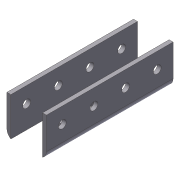
# Autodesk Inventor part: Frame_OuterConveyorMount
Saved by Autodesk Inventor 2012 (Build 160160000, 160)
## iProperties
Created: 2012-01-13
Part Number: Frame_OuterConveyorMount
Material: Aluminum-6061
Document SubType Name: Modeling
Designer: JesseK
Density: 2.71 g/cm^3
Mass: 57.9828 g
Surface Area: 157.919 cm^2
Volume: 21.3958 cm^3
Author: JesseK
Autodesk Inventor part; units mm, degrees
ref_plane "YZ Plane" through (0, 0, 0) normal (1, 0, 0) x (0, 1, 0)
ref_plane "XZ Plane" through (0, 0, 0) normal (0, 1, 0) x (-1, 0, 0)
ref_plane "XY Plane" through (0, 0, 0) normal (0, 0, 1) x (1, 0, 0)
sketch "Sketch1" plane through (0, 0, 0) normal (0, 0, 1) x (1, 0, 0)
  line L0 (0, 25.4) -> (0, 0)
  line L1 (6.35, -6.35) -> (25.4, -6.35)
  line L2 (31.75, 0) -> (31.75, 25.4)
  line L3 (31.75, 25.4) -> (28.575, 25.4)
  line L4 (28.575, 25.4) -> (28.575, 0)
  line L5 (25.4, -3.175) -> (6.35, -3.175)
  line L6 (3.175, 0) -> (3.175, 25.4)
  line L7 (3.175, 25.4) -> (0, 25.4)
  arc A0 (3.175, 0) -> (6.35, -3.175) centre (6.35, 0) ccw
  arc A1 (0, 0) -> (6.35, -6.35) centre (6.35, 0) ccw
  arc A2 (25.4, -3.175) -> (28.575, 0) centre (25.4, 0) ccw
  arc A3 (25.4, -6.35) -> (31.75, 0) centre (25.4, 0) ccw
  dimension "d0" = 3.175
  dimension "d1" = 25.4
  dimension "d2" = 25.4
  dimension "d3" = 3.175
  constraints: 17 end point, 8 point on circle, 8 tangent, 4 centre point, 4 horizontal, 4 vertical, 2 concentric, 1 coincident, 1 equal radius, 1 parallel
  measures "d0" distance between parallel lines of L6 L0
  measures "d1" distance of L6.start L6.end
  measures "d2" distance between parallel lines of L4 L6
  measures "d3" radius of A0
extrude "Extrusion1" add sketch "Sketch1" along normal blind 101.6
sketch "Sketch2" plane through (31.75, 0, 0) normal (1, 0, 0) x (0, 0, -1)
  line L0 (-101.6, 25.4) -> (-101.6, 0) projected
  line L1 (0, 25.4) -> (-101.6, 25.4) projected
  circle A0 centre (-88.9, 12.7) radius 3.175
  dimension "d6" = 6.35
  dimension "d7" = 12.7
  dimension "d8" = 12.7
  constraints: 1 centre point
  measures "d6" diameter of A0
  measures "d7" distance from line of L0 A0.centre
  measures "d8" distance from line of L1 A0.centre
extrude "Extrusion2" cut sketch "Sketch2" against normal through all
pattern_linear "Rectangular Pattern1" count 7 spacing 25.4 along (0, 0, -1) of "Extrusion2"
sketch "Sketch3" plane through (6.35, -6.35, 0) normal (0, -1, 0) x (1, 0, 0)
  line L0 (19.05, 101.6) -> (0, 101.6) projected
  circle A0 centre (9.525, 50.8) radius 6.35
  point P0 (-6.35, 0)
  dimension "d14" = 12.7
  dimension "d15" = 50.8
  constraints: 1 centre point
  measures "d14" diameter of A0
  measures "d15" distance from line of L0 A0.centre
extrude "Extrusion3" cut sketch "Sketch3" against normal up to next
sketch "Sketch4" plane through (6.35, -6.35, 0) normal (0, -1, 0) x (1, 0, 0)
  line L0 (19.05, 101.6) -> (0, 101.6) projected
  line L1 (0, 0) -> (0, 101.6) projected
  line L2 (0, 0) -> (19.05, 0) projected
  line L3 (19.05, 0) -> (19.05, 101.6) projected
  line L4 (-3.175, 101.6) -> (22.225, 101.6)
  line L5 (22.225, 101.6) -> (22.225, 73.025)
  line L6 (22.225, 73.025) -> (-3.175, 73.025)
  line L7 (-3.175, 73.025) -> (-3.175, 101.6)
  line L8 (-3.175, 165.9576) -> (0, 165.9576) construction
  line L9 (19.05, 165.9576) -> (22.225, 165.9576) construction
  line L10 (-3.175, 0) -> (22.225, 0)
  line L11 (22.225, 0) -> (22.225, 28.575)
  line L12 (22.225, 28.575) -> (-3.175, 28.575)
  line L13 (-3.175, 28.575) -> (-3.175, 0)
  line L14 (-6.35, 101.6) -> (-3.175, 101.6)
  line L15 (-3.175, 101.6) -> (-3.175, 73.025)
  line L16 (-3.175, 73.025) -> (-6.35, 73.025)
  line L17 (-6.35, 73.025) -> (-6.35, 101.6)
  point P0 (-6.35, 0)
  dimension "d18" = 25.4
  dimension "d19" = 28.575
  dimension "d20" = 0
  dimension "d21" = 0
  constraints: 28 end point, 6 parallel, 5 horizontal, 4 collinear, 4 point on line, 3 perpendicular
  measures "d18" distance of L5.end L6.end
  measures "d19" distance of L6.end L4.start
  measures "d20" distance between parallel lines of L0 L4
  measures "d21" distance between parallel lines of L2 L10
extrude "Extrusion4" cut sketch "Sketch4" against normal through all contours L3 L6 L1 L0 | L4 L5 L6 L3 | L1 L6 L7 L4 | L12 L11 L10 L3 | L3 L2 L1 L12 | L1 L10 L13 L12
body "Solid1"
